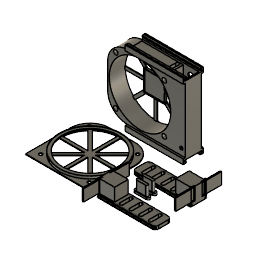
fume_extractor (Autodesk Fusion 360 design; units mm, degrees)
part number: 2026-06-15-13-21-27-474
Autodesk Fusion 360 part; units mm, degrees
(part 1 of 2)
sketch "Sketch1" plane through (0, 0, 0) normal (0, 0, 1) x (1, 0, 0)
  line L0 (-50, -12.5) -> (50, -12.5)
  line L1 (50, -12.5) -> (50, 12.5)
  line L2 (50, 12.5) -> (-50, 12.5)
  line L3 (-50, 12.5) -> (-50, -12.5)
  line L4 (-50, -12.5) -> (50, 12.5) construction
  line L5 (50, -12.5) -> (-50, 12.5) construction
  dimension "d1" = 100
  dimension "d2" = 25
  constraint horizontal L0
  constraint perpendicular L0 L1
  constraint parallel L0 L2
  constraint parallel L1 L3
  constraint coincident L4 origin
  constraint coincident L5 origin
  measures "d1" distance of L1.end L2.end
  measures "d2" distance of L0.end L1.end
extrude "Extrude1" add sketch "Sketch1" along normal blind 120 makes body 1
sketch "Sketch2" plane through (0, 12.5, 0) normal (0, 1, 0) x (-1, 0, 0)
  line L0 (-50, 0) -> (50, 0)
  line L1 (50, 0) -> (50, 120)
  line L2 (50, 120) -> (-50, 120)
  line L3 (-50, 120) -> (-50, 0)
  line L4 (50.0049, 20) -> (-50, 20)
  line L5 (50, 20.0049) -> (50.0049, 20)
  circle A0 centre (0.0025, 70) radius 47.5
  line L6 (6.038, 72.5) -> (47.4366, 72.5)
  line L7 (6.038, 72.5) -> (35.3113, 101.7733)
  line L8 (2.5025, 22.5658) -> (2.5025, 63.9645)
  line L9 (31.7757, 105.3088) -> (2.5025, 76.0355)
  line L10 (-31.7708, 105.3088) -> (-2.4975, 76.0355)
  line L11 (-47.4317, 72.5) -> (-6.0331, 72.5)
  line L12 (-6.0331, 72.5) -> (-35.3063, 101.7733)
  line L13 (47.4366, 67.5) -> (6.038, 67.5)
  line L14 (-6.0331, 67.5) -> (-47.4317, 67.5)
  line L15 (6.038, 67.5) -> (35.3113, 38.2267)
  line L16 (31.7757, 34.6912) -> (2.5025, 63.9645)
  line L17 (-35.3063, 38.2267) -> (-6.0331, 67.5)
  line L18 (-2.4975, 63.9645) -> (-31.7708, 34.6912)
  line L19 (2.5025, 76.0355) -> (2.5025, 117.4342)
  line L20 (-2.4975, 117.4342) -> (-2.4975, 76.0355)
  line L21 (-2.4975, 63.9645) -> (-2.4975, 22.5658)
  point P0 (0.0025, 70)
  point P1 (0.0025, 70)
  point P2 (1.7702, 71.7678)
  dimension "d6" = 20
  dimension "d7" = 95
  constraint coincident L3 L4.end
  constraint parallel L2 L4
  constraint coincident L5 P1
  constraint coincident L1 L5.start
  constraint horizontal L11
  constraint parallel L11 L14
  constraint coincident P1 P0
  constraint parallel L8 L21
  constraint parallel L10 L12
  constraint collinear L20 L21
  constraint collinear L13 L14
  constraint parallel L15 L16
  constraint coincident A0 L12.end
  constraint coincident A0 L10.start
  constraint coincident A0 L11.start
  constraint coincident A0 L14.end
  constraint coincident A0 L19.end
  constraint coincident A0 L20.start
  constraint coincident A0 L9.start
  constraint coincident A0 L7.end
  constraint coincident A0 L6.end
  constraint coincident A0 L13.start
  constraint coincident A0 L15.end
  constraint coincident A0 L16.start
  constraint coincident A0 L21.end
  constraint coincident A0 L8.start
  constraint coincident A0 L17.start
  constraint coincident A0 L18.end
  measures "d6" distance of L0 L4
  measures "d7" diameter of A0
extrude "Extrude2" cut sketch "Sketch2" against normal blind 25 contours A0 L6 L7 | A0 L13 L15 | A0 L9 L19 | A0 L8 L16 | A0 L10 L20 | A0 L18 L21 | A0 L11 L12 | A0 L14 L17 bodies 1
sketch "Sketch7" plane through (0, -12.5, 0) normal (0, -1, 0) x (1, 0, 0)
  line L0 (-50, 0) -> (50, 0)
  line L1 (50, 0) -> (50, 120)
  line L2 (50, 120) -> (-50, 120)
  line L3 (-50, 120) -> (-50, 0)
  line L4 (2.4975, 22.5658) -> (2.4975, 63.9645)
  line L5 (2.4975, 63.9645) -> (31.7708, 34.6912)
  arc A0 (2.4975, 22.5658) -> (31.7708, 34.6912) centre (-0.0025, 70) ccw
  line L6 (-31.7757, 34.6912) -> (-2.5025, 63.9645)
  line L7 (-2.5025, 63.9645) -> (-2.5025, 22.5658)
  arc A1 (-31.7757, 34.6912) -> (-2.5025, 22.5658) centre (-0.0025, 70) ccw
  line L8 (-35.3113, 101.7733) -> (-6.038, 72.5)
  line L9 (-6.038, 72.5) -> (-47.4366, 72.5)
  arc A2 (-35.3113, 101.7733) -> (-47.4366, 72.5) centre (-0.0025, 70) ccw
  line L10 (2.4975, 76.0355) -> (2.4975, 117.4342)
  arc A3 (31.7708, 105.3088) -> (2.4975, 117.4342) centre (-0.0025, 70) ccw
  line L11 (31.7708, 105.3088) -> (2.4975, 76.0355)
  line L12 (-2.5025, 117.4342) -> (-2.5025, 76.0355)
  line L13 (-2.5025, 76.0355) -> (-31.7757, 105.3088)
  arc A4 (-2.5025, 117.4342) -> (-31.7757, 105.3088) centre (-0.0025, 70) ccw
  arc A5 (-47.4366, 67.5) -> (-35.3113, 38.2267) centre (-0.0025, 70) ccw
  line L14 (-47.4366, 67.5) -> (-6.038, 67.5)
  line L15 (-6.038, 67.5) -> (-35.3113, 38.2267)
  line L16 (6.0331, 67.5) -> (47.4317, 67.5)
  arc A6 (35.3063, 38.2267) -> (47.4317, 67.5) centre (-0.0025, 70) ccw
  line L17 (35.3063, 38.2267) -> (6.0331, 67.5)
  arc A7 (47.4317, 72.5) -> (35.3063, 101.7733) centre (-0.0025, 70) ccw
  line L18 (47.4317, 72.5) -> (6.0331, 72.5)
  line L19 (6.0331, 72.5) -> (35.3063, 101.7733)
  circle A8 centre (-0.0025, 70) radius 47.5
  dimension "d36" = 95
  constraint concentric A0 A8
  measures "d36" diameter of A8
extrude "Extrude7" cut sketch "Sketch7" against normal blind 24 contours L4 L5 L6 L7 L8 L9 L10 L11 L12 L13 L14 L15 L16 L17 L18 L19 A8 bodies 1
sketch "Sketch8" plane through (0, 11.5, 0) normal (0, -1, 0) x (1, 0, 0)
  arc A0 (47.4317, 67.5) -> (47.4317, 72.5) centre (-0.0025, 70) ccw
  line L0 (47.4317, 72.5) -> (6.0331, 72.5)
  line L1 (6.0331, 72.5) -> (35.3063, 101.7733)
  arc A1 (35.3063, 101.7733) -> (31.7708, 105.3088) centre (-0.0025, 70) ccw
  line L2 (31.7708, 105.3088) -> (2.4975, 76.0355)
  line L3 (2.4975, 76.0355) -> (2.4975, 117.4342)
  arc A2 (2.4975, 117.4342) -> (-2.5025, 117.4342) centre (-0.0025, 70) ccw
  line L4 (-2.5025, 117.4342) -> (-2.5025, 76.0355)
  line L5 (-2.5025, 76.0355) -> (-31.7757, 105.3088)
  arc A3 (-31.7757, 105.3088) -> (-35.3113, 101.7733) centre (-0.0025, 70) ccw
  line L6 (-35.3113, 101.7733) -> (-6.038, 72.5)
  line L7 (-6.038, 72.5) -> (-47.4366, 72.5)
  arc A4 (-47.4366, 72.5) -> (-47.4366, 67.5) centre (-0.0025, 70) ccw
  line L8 (-47.4366, 67.5) -> (-6.038, 67.5)
  line L9 (-6.038, 67.5) -> (-35.3113, 38.2267)
  arc A5 (-35.3113, 38.2267) -> (-31.7757, 34.6912) centre (-0.0025, 70) ccw
  line L10 (-31.7757, 34.6912) -> (-2.5025, 63.9645)
  line L11 (-2.5025, 63.9645) -> (-2.5025, 22.5658)
  arc A6 (-2.5025, 22.5658) -> (2.4975, 22.5658) centre (-0.0025, 70) ccw
  line L12 (2.4975, 22.5658) -> (2.4975, 63.9645)
  line L13 (2.4975, 63.9645) -> (31.7708, 34.6912)
  arc A7 (31.7708, 34.6912) -> (35.3063, 38.2267) centre (-0.0025, 70) ccw
  line L14 (35.3063, 38.2267) -> (6.0331, 67.5)
  line L15 (6.0331, 67.5) -> (47.4317, 67.5)
  line L16 (16.4975, 86.5) -> (-16.5025, 86.5)
  line L17 (-16.5025, 86.5) -> (-16.5025, 53.5)
  line L18 (-16.5025, 53.5) -> (16.4975, 53.5)
  line L19 (16.4975, 53.5) -> (16.4975, 86.5)
  line L20 (16.4975, 86.5) -> (-16.5025, 53.5) construction
  line L21 (-16.5025, 86.5) -> (16.4975, 53.5) construction
  point P0 (-0.0025, 70)
  dimension "d39" = 33
  dimension "d40" = 33
  constraint horizontal L16
  constraint perpendicular L16 L17
  constraint parallel L16 L18
  constraint parallel L17 L19
  constraint coincident L20 P0
  constraint coincident L21 P0
  constraint coincident P0 A0.centre
  measures "d39" distance of L17.end L18.end
  measures "d40" distance of L16.end L17.end
extrude "Extrude8" add sketch "Sketch8" along normal blind 2 contours L14 L15 L19 | L0 L1 L2 L3 L4 L5 L6 L7 L8 L9 L10 L11 L12 L13 L14 L15 L16 L17 L18 L19 | L0 L1 L19 | L12 L13 L18 | L2 L3 L16 | L10 L11 L18 | L4 L5 L16 | L8 L9 L17 | L6 L7 L17 bodies 1
extrude "Extrude9" add 8 faces at (-13.0143, 11.5, 64.0118) (-13.0143, 11.5, 75.9882) (-5.9906, 11.5, 83.0118) (5.9857, 11.5, 83.0118) (13.0094, 11.5, 75.9882) (13.0094, 11.5, 64.0118) (5.9857, 11.5, 56.9882) (-5.9906, 11.5, 56.9882) along direction (0, 1, 0) blind 1 on bodies 1 bodies 1
sketch "Sketch9" plane through (0, 9.5, 0) normal (0, -1, 0) x (1, 0, 0)
  line L0 (16.4975, 53.5) -> (16.4975, 86.5)
  line L1 (16.4975, 86.5) -> (-16.5025, 86.5)
  line L2 (-16.5025, 86.5) -> (-16.5025, 53.5)
  line L3 (-16.5025, 53.5) -> (16.4975, 53.5)
  line L4 (15.4975, 85.5) -> (-15.5025, 85.5)
  line L5 (-15.5025, 85.5) -> (-15.5025, 54.5)
  line L6 (-15.5025, 54.5) -> (15.4975, 54.5)
  line L7 (15.4975, 54.5) -> (15.4975, 85.5)
  dimension "d45" = 31
  dimension "d46" = 31
  constraint horizontal L4
  constraint perpendicular L4 L5
  constraint parallel L4 L6
  constraint parallel L5 L7
  measures "d45" distance of L5.end L6.end
  measures "d46" distance of L4.end L5.end
extrude "Extrude10" cut sketch "Sketch9" against normal blind 1 contours L4 L5 L6 L7 bodies 1
sketch "Sketch10" plane through (0, 9.5, 0) normal (0, -1, 0) x (1, 0, 0)
  line L0 (-15.5025, 85.5) -> (15.4975, 85.5)
  line L1 (15.4975, 85.5) -> (15.4975, 54.5)
  line L2 (15.4975, 54.5) -> (-15.5025, 54.5)
  line L3 (-15.5025, 54.5) -> (-15.5025, 85.5)
  line L4 (16.4975, 53.5) -> (16.4975, 86.5)
  line L5 (16.4975, 86.5) -> (-16.5025, 86.5)
  line L6 (-16.5025, 86.5) -> (-16.5025, 53.5)
  line L7 (-16.5025, 53.5) -> (16.4975, 53.5)
  line L8 (-1.5, 53.5) -> (-1.5, 54.5)
  line L9 (1.5, 54.5) -> (1.5, 53.5)
  constraint coincident L7 L8.start
  constraint coincident L2 L8.end
  constraint perpendicular L2 L8
  constraint coincident L2 L9.start
  constraint coincident L7 L9.end
  constraint perpendicular L7 L9
extrude "Extrude11" cut sketch "Sketch10" against normal blind 2 contours L2 L7 L8 L9 bodies 1
fillet "Fillet1" radius 30 1 edges at (-50, 0, 120) on bodies 1
fillet "Fillet2" radius 30 1 edges at (50, 0, 120) on bodies 1
sketch "Sketch3" plane through (50, 0, 0) normal (1, 0, 0) x (0, 1, 0)
  line L0 (12.5, 90) -> (-12.5, 90)
  line L1 (-12.5, 90) -> (-12.5, 0)
  line L2 (-12.5, 0) -> (12.5, 0)
  line L3 (12.5, 0) -> (12.5, 90)
  line L4 (-10.5, 20) -> (10.5, 20)
  line L5 (10.5, 20) -> (10.5, 2)
  line L6 (10.5, 2) -> (-10.5, 2)
  line L7 (-10.5, 2) -> (-10.5, 20)
  dimension "d14" = 2
  dimension "d15" = 2
  dimension "d16" = 2
  dimension "d17" = 18
  constraint horizontal L4
  constraint vertical L5
  constraint horizontal L6
  constraint vertical L7
  measures "d14" distance of L3 L5
  measures "d15" distance of L1 L7
  measures "d16" distance of L2 L6
  measures "d17" distance of L4 L6
extrude "Extrude3" cut sketch "Sketch3" against normal blind 98 contours L4 L5 L6 L7 bodies 1
sketch "Sketch4" plane through (0, -10.5, 0) normal (0, 1, 0) x (-1, 0, 0)
  line L0 (-50, 20) -> (-50, 2)
  line L1 (-50, 2) -> (48, 2)
  line L2 (48, 2) -> (48, 20)
  line L3 (48, 20) -> (-50, 20)
  circle A0 centre (-41, 14.5) radius 4.5
  dimension "d20" = 9
  dimension "d21" = 9
  dimension "d22" = 12.5
  measures "d20" diameter of A0
  measures "d21" distance of L0 A0.centre
  measures "d22" distance of L1 A0.centre
extrude "Extrude4" cut sketch "Sketch4" along normal blind 33 contours A0 bodies 1
sketch "Sketch6" plane through (0, 0, 20) normal (0, 0, -1) x (1, 0, 0)
  line L0 (50, -10.5) -> (50, 10.5)
  line L1 (50, 10.5) -> (-48, 10.5)
  line L2 (-48, 10.5) -> (-48, -10.5)
  line L3 (-48, -10.5) -> (50, -10.5)
  circle A0 centre (0, -1.1091) radius 2.5
  dimension "d27" = 5
  measures "d27" diameter of A0
extrude "Extrude6" cut sketch "Sketch6" against normal blind 50 contours A0 bodies 1
sketch "Sketch5" plane through (50, 0, 0) normal (1, 0, 0) x (0, 1, 0)
  line L0 (10.5, 20) -> (10.5, 2)
  line L1 (10.5, 2) -> (-10.5, 2)
  line L2 (-10.5, 2) -> (-10.5, 20)
  line L3 (-10.5, 20) -> (10.5, 20)
  line L4 (12.5, 90) -> (-12.5, 90)
  line L5 (-12.5, 90) -> (-12.5, 0)
  line L6 (-12.5, 0) -> (12.5, 0)
  line L7 (12.5, 0) -> (12.5, 90)
  line L8 (10.5, 20) -> (-10.5, 20)
  line L9 (-10.5, 20) -> (-10.5, 26)
  line L10 (-10.5, 26) -> (10.5, 26)
  line L11 (10.5, 26) -> (10.5, 20)
  constraint perpendicular L8 L9
  constraint parallel L8 L10
  constraint parallel L9 L11
  constraint coincident L2.end L3.start
  constraint perpendicular L2 L8
  constraint coincident L0.start L3.end
extrude "Extrude5" cut sketch "Sketch5" against normal blind 20 contours L3 L8 L9 L10 L11 bodies 1
sketch "Sketch12" plane through (0, -12.5, 0) normal (0, -1, 0) x (1, 0, 0)
  circle A0 centre (-0.0025, 70) radius 47.5
  arc A1 (50, 90) -> (20, 120) centre (20, 90) ccw
  line L0 (20, 120) -> (-20, 120)
  arc A2 (-20, 120) -> (-50, 90) centre (-20, 90) ccw
  line L1 (-50, 90) -> (-50, 0)
  line L2 (-50, 0) -> (50, 0)
  line L3 (50, 0) -> (50, 90)
  circle A3 centre (-40, 6) radius 2.5
  dimension "d54" = 5
  measures "d54" diameter of A3
extrude "Extrude13" cut sketch "Sketch12" against normal blind 2 contours A3 bodies 1
sketch "Sketch13" plane through (0, -12.5, 0) normal (0, -1, 0) x (1, 0, 0)
  circle A0 centre (-40, 6) radius 2.5
  circle A1 centre (-0.0025, 70) radius 47.5
  arc A2 (50, 90) -> (20, 120) centre (20, 90) ccw
  line L0 (20, 120) -> (-20, 120)
  arc A3 (-20, 120) -> (-50, 90) centre (-20, 90) ccw
  line L1 (-50, 90) -> (-50, 0)
  line L2 (-50, 0) -> (50, 0)
  line L3 (50, 0) -> (50, 90)
  line L4 (0, 120) -> (0, 117.5)
  circle A4 centre (37.5, 107.5005) radius 3.5
  circle A5 centre (-37.5, 107.5005) radius 3.5
  circle A6 centre (37.5, 32.5005) radius 3.5
  circle A7 centre (-37.5, 32.5005) radius 3.5
  line L5 (-37.5, 107.5005) -> (37.5, 107.5005)
  line L6 (37.5, 107.5005) -> (37.5, 32.5005)
  line L7 (37.5, 32.5005) -> (-37.5, 32.5005)
  line L8 (-37.5, 32.5005) -> (-37.5, 107.5005)
  dimension "d59" = 75
  dimension "d63" = 75
  dimension "d64" = 37.5
  dimension "d67" = 7
  dimension "d68" = 7
  dimension "d69" = 7
  dimension "d70" = 7
  dimension "d71" = 75
  constraint midpoint L0 L4.start
  constraint perpendicular L0 L4
  constraint coincident A1 L4.end
  constraint coincident A5.centre L5.start
  constraint coincident A4.centre L5.end
  constraint horizontal L5
  constraint coincident A6.centre L6.end
  constraint perpendicular L5 L6
  constraint coincident A7.centre L7.end
  constraint perpendicular L6 L7
  measures "d59" distance of A4.centre A5.centre
  measures "d63" horizontal distance of A6.centre A7.centre
  measures "d64" distance of L4 A5.centre
  measures "d67" diameter of A4
  measures "d68" diameter of A5
  measures "d69" diameter of A6
  measures "d70" diameter of A7
  measures "d71" distance of A5.centre A7.centre
extrude "Extrude14" cut sketch "Sketch13" against normal blind 6 contours A4 L5 L6 | A4 L5 L6 | A6 L6 L7 | A6 L6 L7 | A5 L5 L8 | A5 L5 L8 | A7 L7 L8 | A7 L7 L8 bodies 1
sketch "Sketch14" plane through (0, 0, 0) normal (0, 0, 1) x (1, 0, 0)
  line L0 (20, 50) -> (-20, 50)
  line L1 (-50, 20) -> (-50, -50)
  line L2 (-50, -50) -> (50, -50)
  line L3 (50, -50) -> (50, 20)
  arc A0 (-20, 50) -> (-50, 20) centre (-20, 20) ccw
  arc A1 (50, 20) -> (20, 50) centre (20, 20) ccw
  circle A2 centre (0, 0) radius 47.5
  line L4 (-50, 50) -> (-41.2132, 41.2132) construction
  line L5 (50, 50) -> (41.2132, 41.2132) construction
  circle A3 centre (-37.7911, 36.5) radius 2.5
  circle A4 centre (37.2089, 36.5) radius 2.5
  circle A5 centre (-37.7911, -38.5) radius 2.5
  circle A6 centre (37.2089, -38.5) radius 2.5
  dimension "d72" = 100
  dimension "d73" = 100
  dimension "d74" = 30
  dimension "d75" = 30
  dimension "d76" = 95
  dimension "d81" = 75
  dimension "d82" = 75
  dimension "d84" = 50
  dimension "d85" = 5
  dimension "d86" = 5
  dimension "d87" = 5
  dimension "d88" = 5
  constraint horizontal L0
  constraint perpendicular L0 L1
  constraint parallel L0 L2
  constraint parallel L1 L3
  constraint coincident A2.centre origin
  constraint coincident L4.start L0
  constraint coincident L4.start L1
  constraint tangent L0 A0
  constraint tangent L1 A0
  constraint coincident L5.start L0
  constraint coincident L5.start L3
  constraint tangent L0 A1
  constraint tangent L3 A1
  constraint coincident A0 L4.end
  constraint coincident A1 L5.end
  measures "d72" distance of L1.end L2.end
  measures "d73" distance of L4.start L1.end
  measures "d74" radius of A0
  measures "d75" radius of A1
  measures "d76" diameter of A2
  measures "d81" distance of A3.centre A4.centre
  measures "d82" vertical distance of A3.centre A5.centre
  measures "d84" distance of L0 A2.centre
  measures "d85" diameter of A3
  measures "d86" diameter of A4
  measures "d87" diameter of A5
  measures "d88" diameter of A6
extrude "Extrude15" add sketch "Sketch14" along normal blind 1 separate body makes body 2
sketch "Sketch15" plane through (0, 0, 0) normal (0, 0, 1) x (1, 0, 0)
  circle A0 centre (0, 0) radius 46.5
  circle A1 centre (0, 0) radius 47.5
  dimension "d91" = 93
  dimension "d92" = 95
  constraint coincident A0.centre A1.centre
  constraint concentric A0 A1
  measures "d91" diameter of A0
  measures "d92" diameter of A1
extrude "Extrude16" add sketch "Sketch15" along normal blind 5 bodies 2
sketch "Sketch16" plane through (0, 0, 0) normal (0, 0, 1) x (1, 0, 0)
  circle A0 centre (0, 0) radius 45
  circle A1 centre (0, 0) radius 46.5
  dimension "d95" = 90
  dimension "d96" = 93
  constraint coincident A0.centre A1.centre
  constraint concentric A0 A1
  measures "d95" diameter of A0
  measures "d96" diameter of A1
extrude "Extrude17" add sketch "Sketch16" along normal blind 1 bodies 2
sketch "Sketch17" plane through (0, 0, 5) normal (0, 0, 1) x (-1, 0, 0)
  circle A0 centre (0, 0) radius 46.5
  circle A1 centre (0, 0) radius 47.5
  circle A2 centre (0, 0) radius 42.5
  circle A3 centre (0.5775, 0) radius 47.0775
  dimension "d99" = 85
  constraint concentric A0 A2
  constraint tangent A0 A3
  measures "d99" diameter of A2
extrude "Extrude18" add sketch "Sketch17" against normal blind 1 contours A0 bodies 2
sketch "Sketch18" plane through (0, 0, 0) normal (0, 0, 1) x (1, 0, 0)
  line L0 (-33.5384, 30.0029) -> (-6.0355, 2.5)
  line L1 (6.0355, 2.5) -> (33.5384, 30.0029)
  line L2 (30.0029, 33.5384) -> (2.5, 6.0355)
  line L3 (6.0355, -2.5) -> (33.5384, -30.0029)
  line L4 (30.0029, -33.5384) -> (2.5, -6.0355)
  line L5 (-30.0029, -33.5384) -> (-2.5, -6.0355)
  line L6 (-6.0355, -2.5) -> (-33.5384, -30.0029)
  line L7 (-2.5, 6.0355) -> (-30.0029, 33.5384)
  line L8 (44.9305, 2.5) -> (6.0355, 2.5)
  line L9 (-6.0355, 2.5) -> (-44.9305, 2.5)
  line L10 (-44.9305, -2.5) -> (-6.0355, -2.5)
  line L11 (6.0355, -2.5) -> (44.9305, -2.5)
  line L12 (2.5, 6.0355) -> (2.5, 44.9305)
  line L13 (2.5, -44.9305) -> (2.5, -6.0355)
  line L14 (-2.5, 44.9305) -> (-2.5, 6.0355)
  line L15 (-2.5, -6.0355) -> (-2.5, -44.9305)
  arc A0 (-44.9305, 2.5) -> (-44.9305, -2.5) centre (0, 0) ccw
  arc A1 (-30.0029, 33.5384) -> (-33.5384, 30.0029) centre (0, 0) ccw
  arc A2 (2.5, 44.9305) -> (-2.5, 44.9305) centre (0, 0) ccw
  arc A3 (33.5384, 30.0029) -> (30.0029, 33.5384) centre (0, 0) ccw
  arc A4 (44.9305, -2.5) -> (44.9305, 2.5) centre (0, 0) ccw
  arc A5 (30.0029, -33.5384) -> (33.5384, -30.0029) centre (0, 0) ccw
  arc A6 (-33.5384, -30.0029) -> (-30.0029, -33.5384) centre (0, 0) ccw
  arc A7 (-2.5, -44.9305) -> (2.5, -44.9305) centre (0, 0) ccw
  constraint horizontal L10
  constraint parallel L8 L11
  constraint coincident A0.centre A1.centre
  constraint parallel L13 L15
  constraint parallel L0 L7
  constraint parallel L1 L2
  constraint parallel L3 L4
  constraint collinear L8 L9
  constraint collinear L10 L11
  constraint collinear L14 L15
  constraint concentric A0 A6
  constraint concentric A1 A2
  constraint concentric A2 A3
  constraint concentric A3 A4
  constraint concentric A4 A5
  constraint concentric A5 A7
  constraint concentric A6 A7
extrude "Extrude19" add sketch "Sketch18" along normal blind 1 bodies 2
move_body "Move2" bodies 2 to x (1, 0, 0) y (0, 1, 0) z (0, 0, 1) at (-1.2204, -73.9859, 0)
sketch "Sketch19" plane through (0, 0, 0) normal (0, 0, 1) x (1, 0, 0)
  line L0 (51.3826, -12.4971) -> (56.3826, -12.4971)
  line L1 (56.3826, -12.4971) -> (56.3826, 12.5029)
  line L2 (56.3826, 12.5029) -> (51.3826, 12.5029)
  line L3 (51.3826, 12.5029) -> (51.3826, -12.4971)
  dimension "d108" = 5
  dimension "d113" = 25
  constraint horizontal L0
  constraint vertical L1
  constraint horizontal L2
  constraint vertical L3
  measures "d108" distance of L0.start L0.end
  measures "d113" distance of L0.end L1.end
extrude "Extrude20" add sketch "Sketch19" along normal blind 90 separate body makes body 3
sketch "Sketch21" plane through (56.3826, 0, 0) normal (1, 0, 0) x (0, 1, 0)
  line L0 (-12.4971, 0) -> (12.5029, 0)
  line L1 (12.5029, 0) -> (12.5029, 90)
  line L2 (12.5029, 90) -> (-12.4971, 90)
  line L3 (-12.4971, 90) -> (-12.4971, 0)
  line L4 (7.5, 80) -> (-7.5, 80)
  line L5 (-7.5, 75) -> (7.5, 75)
  line L6 (7.5, 65) -> (-7.5, 65)
  line L7 (-7.5, 60) -> (7.5, 60)
  line L8 (7.5, 50) -> (-7.5, 50)
  line L9 (-7.5, 45) -> (7.5, 45)
  line L10 (7.5, 35) -> (-7.5, 35)
  line L11 (-7.5, 30) -> (7.5, 30)
  arc A0 (7.5, 75) -> (7.5, 80) centre (7.5, 77.5) ccw
  arc A1 (-7.5, 80) -> (-7.5, 75) centre (-7.5, 77.5) ccw
  arc A2 (-7.5, 65) -> (-7.5, 60) centre (-7.5, 62.5) ccw
  arc A3 (7.5, 60) -> (7.5, 65) centre (7.5, 62.5) ccw
  arc A4 (-7.5, 50) -> (-7.5, 45) centre (-7.5, 47.5) ccw
  arc A5 (7.5, 45) -> (7.5, 50) centre (7.5, 47.5) ccw
  arc A6 (-7.5, 35) -> (-7.5, 30) centre (-7.5, 32.5) ccw
  arc A7 (7.5, 30) -> (7.5, 35) centre (7.5, 32.5) ccw
  dimension "d116" = 10
  dimension "d119" = 10
  dimension "d124" = 10
  dimension "d125" = 10
  dimension "d126" = 2.5
  dimension "d127" = 2.5
  dimension "d128" = 2.5
  constraint horizontal L4
  constraint parallel L4 L5
  constraint horizontal L6
  constraint parallel L6 L7
  constraint horizontal L8
  constraint parallel L8 L9
  constraint horizontal L10
  constraint parallel L10 L11
  constraint tangent L4 A0
  constraint tangent L5 A0
  constraint tangent L6 A2
  constraint tangent L7 A2
  constraint tangent L6 A3
  constraint tangent L7 A3
  constraint tangent L8 A4
  constraint tangent L9 A4
  constraint equal A2 A4
  constraint tangent L8 A5
  constraint tangent L9 A5
  constraint tangent L10 A6
  constraint tangent L11 A6
  constraint equal A2 A6
  constraint tangent L10 A7
  constraint tangent L11 A7
  measures "d116" distance of L2 L4
  measures "d119" distance of L5 L6
  measures "d124" distance of L7 L8
  measures "d125" distance of L9 L10
  measures "d126" radius of A0
  measures "d127" radius of A1
  measures "d128" radius of A2
extrude "Extrude22" cut sketch "Sketch21" against normal blind 5 contours L4 L5 A0 A1 | L6 L7 A2 A3 | L8 L9 A4 A5 | L10 L11 A6 A7 bodies 3
sketch "Sketch22" plane through (50, 0, 0) normal (1, 0, 0) x (0, 1, 0)
  line L0 (12.5, 90) -> (-12.5, 90)
  line L1 (-12.5, 90) -> (-12.5, 0)
  line L2 (-12.5, 0) -> (12.5, 0)
  line L3 (12.5, 0) -> (12.5, 90)
  line L4 (-10.5, 2) -> (-10.5, 26)
  line L5 (-10.5, 26) -> (10.5, 26)
  line L6 (10.5, 26) -> (10.5, 2)
  line L7 (10.5, 2) -> (-10.5, 2)
  line L8 (7.5, 34.5) -> (-7.5, 34.5)
  line L9 (-7.5, 29.5) -> (7.5, 29.5)
  arc A0 (7.5, 29.5) -> (7.5, 34.5) centre (7.5, 32) ccw
  arc A1 (-7.5, 34.5) -> (-7.5, 29.5) centre (-7.5, 32) ccw
  dimension "d133" = 2.5
  constraint horizontal L8
  constraint parallel L8 L9
  constraint tangent L8 A1
  constraint tangent L9 A1
  constraint equal A0 A1
  measures "d133" radius of A0
extrude "Extrude23" cut sketch "Sketch22" against normal blind 7 contours L8 L9 A0 A1 bodies 1
fillet "Fillet3" radius 5 1 edges at (53.8826, -12.4971, 90) on bodies 3
fillet "Fillet4" radius 5 1 edges at (53.8826, 12.5029, 90) on bodies 3
sketch "Sketch23" plane through (56.3826, 0, 0) normal (1, 0, 0) x (0, 1, 0)
  line L0 (-7.5, 65) -> (7.5, 65)
  arc A0 (7.5, 60) -> (7.5, 65) centre (7.5, 62.5) ccw
  line L1 (7.5, 60) -> (-7.5, 60)
  arc A1 (-7.5, 65) -> (-7.5, 60) centre (-7.5, 62.5) ccw
  line L2 (-7.5, 50) -> (7.5, 50)
  arc A2 (7.5, 45) -> (7.5, 50) centre (7.5, 47.5) ccw
  line L3 (7.5, 45) -> (-7.5, 45)
  arc A3 (-7.5, 50) -> (-7.5, 45) centre (-7.5, 47.5) ccw
  line L4 (7.5, 75) -> (-7.5, 75)
  arc A4 (-7.5, 80) -> (-7.5, 75) centre (-7.5, 77.5) ccw
  line L5 (-7.5, 80) -> (7.5, 80)
  arc A5 (7.5, 75) -> (7.5, 80) centre (7.5, 77.5) ccw
  line L6 (-7.5, 35) -> (7.5, 35)
  arc A6 (7.5, 30) -> (7.5, 35) centre (7.5, 32.5) ccw
  line L7 (7.5, 30) -> (-7.5, 30)
  arc A7 (-7.5, 35) -> (-7.5, 30) centre (-7.5, 32.5) ccw
  arc A8 (12.5029, 85) -> (7.5029, 90) centre (7.5029, 85) ccw
  line L8 (7.5029, 90) -> (-7.4971, 90)
  arc A9 (-7.4971, 90) -> (-12.4971, 85) centre (-7.4971, 85) ccw
  line L9 (-12.4971, 85) -> (-12.4971, 0)
  line L10 (-12.4971, 0) -> (12.5029, 0)
  line L11 (12.5029, 0) -> (12.5029, 85)
  line L12 (-12.4971, 0) -> (12.5029, 0)
  line L13 (12.5029, 0) -> (12.5029, 25)
  line L14 (12.5029, 25) -> (-12.4971, 25)
  line L15 (-12.4971, 25) -> (-12.4971, 0)
  dimension "d140" = 25
  constraint perpendicular L12 L13
  constraint parallel L12 L14
  constraint parallel L13 L15
  constraint coincident L10.end L11.start
  constraint perpendicular L11 L12
  constraint coincident L9.end L10.start
  measures "d140" distance of L9.end L14.end
extrude "Extrude24" add sketch "Sketch23" along normal blind 20 contours L9 L10 L11 L12 L13 L14 L15 bodies 3
sketch "Sketch28" plane through (76.3826, 0, 0) normal (1, 0, 0) x (0, 1, 0)
  line L0 (-12.4971, 25) -> (-12.4971, 0)
  line L1 (-12.4971, 0) -> (12.5029, 0)
  line L2 (12.5029, 0) -> (12.5029, 25)
  line L3 (12.5029, 25) -> (-12.4971, 25)
  line L4 (-10.4971, 25) -> (-10.4971, 2)
  line L5 (-10.4971, 2) -> (10.5029, 2)
  line L6 (10.5029, 2) -> (10.5029, 25)
  constraint coincident L3 L4.start
  constraint perpendicular L1 L4
  constraint perpendicular L2 L5
  constraint coincident L3 L6.end
  constraint perpendicular L3 L6
extrude "Extrude29" cut sketch "Sketch28" against normal blind 20 contours L0 L1 L2 L3 L4 L5 L6 bodies 3
sketch "Sketch29" plane through (56.3826, 0, 0) normal (1, 0, 0) x (0, 1, 0)
  line L0 (12.5029, 0) -> (12.5029, 85)
  line L1 (7.5029, 90) -> (-7.4971, 90)
  arc A0 (-7.4971, 90) -> (-12.4971, 85) centre (-7.4971, 85) ccw
  line L2 (-12.4971, 85) -> (-12.4971, 0)
  line L3 (-12.4971, 0) -> (12.5029, 0)
  line L4 (10.5029, 2) -> (-10.4971, 2)
  line L5 (-10.4971, 2) -> (-10.4971, 25)
  line L6 (-10.4971, 25) -> (10.5029, 25)
  line L7 (-7.5, 65) -> (7.5, 65)
  arc A1 (7.5, 60) -> (7.5, 65) centre (7.5, 62.5) ccw
  line L8 (7.5, 60) -> (-7.5, 60)
  arc A2 (-7.5, 65) -> (-7.5, 60) centre (-7.5, 62.5) ccw
  line L9 (-7.5, 50) -> (7.5, 50)
  arc A3 (7.5, 45) -> (7.5, 50) centre (7.5, 47.5) ccw
  line L10 (7.5, 45) -> (-7.5, 45)
  arc A4 (-7.5, 50) -> (-7.5, 45) centre (-7.5, 47.5) ccw
  line L11 (7.5, 75) -> (-7.5, 75)
  arc A5 (-7.5, 80) -> (-7.5, 75) centre (-7.5, 77.5) ccw
  line L12 (-7.5, 80) -> (7.5, 80)
  arc A6 (7.5, 75) -> (7.5, 80) centre (7.5, 77.5) ccw
  line L13 (-7.5, 35) -> (7.5, 35)
  arc A7 (7.5, 30) -> (7.5, 35) centre (7.5, 32.5) ccw
  line L14 (7.5, 30) -> (-7.5, 30)
  arc A8 (-7.5, 35) -> (-7.5, 30) centre (-7.5, 32.5) ccw
  line L15 (-0.4971, 2) -> (-0.4971, 0)
  line L16 (0.5029, 2) -> (0.5029, 0)
  arc A9 (12.5029, 85) -> (7.5029, 90) centre (7.5029, 85) ccw
  line L17 (10.5029, 25) -> (10.5029, 2)
  dimension "d169" = 12
  dimension "d170" = 12
  constraint coincident L4 L15.start
  constraint coincident L3 L15.end
  constraint perpendicular L3 L15
  constraint coincident L4 L16.start
  constraint coincident L3 L16.end
  constraint perpendicular L3 L16
  measures "d169" distance of L0 L16
  measures "d170" distance of L2 L15
extrude "Extrude30" add sketch "Sketch29" along normal blind 20 contours L3 L4 L15 L16 bodies 3
sketch "Sketch30" plane through (56.3826, 0, 0) normal (1, 0, 0) x (0, 1, 0)
  line L0 (-7.5, 35) -> (7.5, 35)
  arc A0 (7.5, 30) -> (7.5, 35) centre (7.5, 32.5) ccw
  line L1 (7.5, 30) -> (-7.5, 30)
  arc A1 (-7.5, 35) -> (-7.5, 30) centre (-7.5, 32.5) ccw
  line L2 (7.5, 75) -> (-7.5, 75)
  arc A2 (-7.5, 80) -> (-7.5, 75) centre (-7.5, 77.5) ccw
  line L3 (-7.5, 80) -> (7.5, 80)
  arc A3 (7.5, 75) -> (7.5, 80) centre (7.5, 77.5) ccw
  line L4 (-7.5, 50) -> (7.5, 50)
  arc A4 (7.5, 45) -> (7.5, 50) centre (7.5, 47.5) ccw
  line L5 (7.5, 45) -> (-7.5, 45)
  arc A5 (-7.5, 50) -> (-7.5, 45) centre (-7.5, 47.5) ccw
  line L6 (-7.5, 65) -> (7.5, 65)
  arc A6 (7.5, 60) -> (7.5, 65) centre (7.5, 62.5) ccw
  line L7 (7.5, 60) -> (-7.5, 60)
  arc A7 (-7.5, 65) -> (-7.5, 60) centre (-7.5, 62.5) ccw
  line L8 (-0.4971, 2) -> (-10.4971, 2)
  line L9 (-10.4971, 2) -> (-10.4971, 25)
  line L10 (-10.4971, 25) -> (10.5029, 25)
  line L11 (0.5029, 2) -> (0.5029, 0)
  line L12 (0.5029, 0) -> (12.5029, 0)
  line L13 (12.5029, 0) -> (12.5029, 85)
  line L14 (7.5029, 90) -> (-7.4971, 90)
  arc A8 (-7.4971, 90) -> (-12.4971, 85) centre (-7.4971, 85) ccw
  line L15 (-12.4971, 85) -> (-12.4971, 0)
  line L16 (12.5029, 0) -> (0.5029, 0)
  line L17 (0.5029, 0) -> (0.5029, 2)
  line L18 (0.5029, 2) -> (12.5029, 2)
  line L19 (12.5029, 2) -> (12.5029, 0)
  line L20 (0.5039, 1.5) -> (12.0029, 1.5)
  line L21 (12.0029, 1.5) -> (12.0029, 0.5)
  line L22 (12.0029, 0.5) -> (0.5039, 0.5)
  line L23 (0.5039, 0.5) -> (0.5039, 1.5)
  line L24 (-0.4971, 0) -> (-0.4971, 2)
  line L25 (10.5029, 25) -> (10.5029, 2)
  line L26 (10.5029, 2) -> (0.5029, 2)
  arc A9 (12.5029, 85) -> (7.5029, 90) centre (7.5029, 85) ccw
  line L27 (-12.4971, 0) -> (-0.4971, 0)
  dimension "d173" = 0.5
  dimension "d174" = 0.5
  dimension "d175" = 0.001
  dimension "d176" = 0.5
  constraint horizontal L16
  constraint vertical L17
  constraint horizontal L18
  constraint vertical L19
  constraint coincident L11.start L17.end
  constraint coincident L12.end L13.start
  constraint horizontal L20
  constraint vertical L21
  constraint horizontal L22
  constraint vertical L23
  measures "d173" distance of L16 L22
  measures "d174" distance of L18 L20
  measures "d175" distance of L17 L23
  measures "d176" distance of L19 L20.end
extrude "Extrude31" add sketch "Sketch30" along normal blind 20 contours L11 L12 L13 L16 L17 L18 L19 L26 bodies 3
sketch "Sketch31" plane through (0, 12.5029, 0) normal (0, 1, 0) x (-1, 0, 0)
  line L0 (-76.3826, 0) -> (-51.3826, 0)
  line L1 (-51.3826, 0) -> (-51.3826, 85)
  line L2 (-56.3826, 85) -> (-56.3826, 2)
  line L3 (-76.3826, 2) -> (-76.3826, 0)
  line L4 (-75.8826, 2) -> (-56.8826, 2)
  line L5 (-56.8826, 2) -> (-56.8826, 0)
  line L6 (-56.8826, 0) -> (-75.8826, 0)
  line L7 (-75.8826, 0) -> (-75.8826, 2)
  line L8 (-51.3826, 85) -> (-56.3826, 85)
  line L9 (-56.3826, 2) -> (-76.3826, 2)
  dimension "d179" = 0.5
  dimension "d180" = 5.5
  constraint horizontal L4
  constraint vertical L5
  constraint horizontal L6
  constraint vertical L7
  constraint coincident L0 L5.end
  measures "d179" distance of L3 L7
  measures "d180" distance of L1 L5
extrude "Extrude32" cut sketch "Sketch31" against normal blind 12 contours L0 L4 L5 L6 L7 L9 bodies 3
extrude "Extrude33" add 1 faces at (69.5492, 0.5029, 0.6667) along direction (0, 1, 0) blind 0.001 on bodies 3 bodies 3
extrude "Extrude34" add 1 faces at (69.5492, 0.5039, 0.8333) along direction (0, 1, 0) blind 5 on bodies 3 bodies 3
sketch "Sketch33" plane through (56.3826, 0, 0) normal (1, 0, 0) x (0, 1, 0)
  line L0 (12.5029, 2) -> (12.5029, 85)
  line L1 (-12.4971, 0) -> (-0.4971, 0)
  line L2 (-0.4971, 0) -> (-0.4971, 2)
  line L3 (-0.4971, 2) -> (-10.4971, 2)
  line L4 (-0.4981, 0.5) -> (-11.9971, 0.5)
  line L5 (-11.9971, 0.5) -> (-11.9971, 1.5)
  line L6 (-11.9971, 1.5) -> (-0.4981, 1.5)
  line L7 (-0.4981, 1.5) -> (-0.4981, 0.5)
  line L8 (-10.4971, 2) -> (-12.4971, 2)
  line L9 (10.5029, 2) -> (12.5029, 2)
  arc A0 (12.5029, 85) -> (7.5029, 90) centre (7.5029, 85) ccw
  line L10 (7.5029, 90) -> (-7.4971, 90)
  arc A1 (-7.4971, 90) -> (-12.4971, 85) centre (-7.4971, 85) ccw
  line L11 (-12.4971, 85) -> (-12.4971, 0)
  line L12 (-10.4971, 2) -> (-10.4971, 25)
  line L13 (-10.4971, 25) -> (10.5029, 25)
  line L14 (10.5029, 25) -> (10.5029, 2)
  line L15 (-7.5, 65) -> (7.5, 65)
  arc A2 (7.5, 60) -> (7.5, 65) centre (7.5, 62.5) ccw
  line L16 (7.5, 60) -> (-7.5, 60)
  arc A3 (-7.5, 65) -> (-7.5, 60) centre (-7.5, 62.5) ccw
  line L17 (-7.5, 50) -> (7.5, 50)
  arc A4 (7.5, 45) -> (7.5, 50) centre (7.5, 47.5) ccw
  line L18 (7.5, 45) -> (-7.5, 45)
  arc A5 (-7.5, 50) -> (-7.5, 45) centre (-7.5, 47.5) ccw
  line L19 (7.5, 75) -> (-7.5, 75)
  arc A6 (-7.5, 80) -> (-7.5, 75) centre (-7.5, 77.5) ccw
  line L20 (-7.5, 80) -> (7.5, 80)
  arc A7 (7.5, 75) -> (7.5, 80) centre (7.5, 77.5) ccw
  line L21 (-7.5, 35) -> (7.5, 35)
  arc A8 (7.5, 30) -> (7.5, 35) centre (7.5, 32.5) ccw
  line L22 (7.5, 30) -> (-7.5, 30)
  arc A9 (-7.5, 35) -> (-7.5, 30) centre (-7.5, 32.5) ccw
  dimension "d188" = 0.5
  dimension "d190" = 0.5
  dimension "d191" = 0.001
  constraint horizontal L4
  constraint vertical L5
  constraint horizontal L6
  constraint vertical L7
  constraint coincident L3.end L8.start
  measures "d188" distance of L3 L6
  measures "d190" distance of L1 L4
  measures "d191" distance of L2 L7
extrude "Extrude35" add sketch "Sketch33" along normal blind 20 contours L1 L2 L3 L8 L11 bodies 3
sketch "Sketch34" plane through (0, -12.4971, 0) normal (0, -1, 0) x (1, 0, 0)
  line L0 (56.3826, 85) -> (51.3826, 85)
  line L1 (51.3826, 85) -> (51.3826, 0)
  line L2 (51.3826, 0) -> (76.3826, 0)
  line L3 (76.3826, 0) -> (76.3826, 2)
  line L4 (56.8826, 2) -> (75.8826, 2)
  line L5 (75.8826, 2) -> (75.8826, 0)
  line L6 (75.8826, 0) -> (56.8826, 0)
  line L7 (56.8826, 0) -> (56.8826, 2)
  line L8 (56.3826, 2) -> (56.3826, 85)
  line L9 (76.3826, 2) -> (56.3826, 2)
  dimension "d194" = 0.5
  dimension "d195" = 5.5
  constraint horizontal L4
  constraint vertical L5
  constraint horizontal L6
  constraint vertical L7
  constraint coincident L2 L5.end
  measures "d194" distance of L3 L5
  measures "d195" distance of L1 L7
extrude "Extrude36" cut sketch "Sketch34" against normal blind 12 contours L2 L4 L5 L6 L7 L9 bodies 3
extrude "Extrude37" add 1 faces at (63.2159, -0.4971, 1.3333) along direction (0, -1, 0) blind 0.001 on bodies 3 bodies 3
extrude "Extrude38" add 1 faces at (63.2159, -0.4981, 1.1667) along direction (0, -1, 0) blind 5 on bodies 3 bodies 3
sketch "Sketch36" plane through (56.8826, 0, 0) normal (1, 0, 0) x (0, 1, 0)
  line L0 (5.5039, 2) -> (5.5039, 1.5)
  line L1 (5.5039, 1.5) -> (12.0029, 1.5)
  line L2 (12.0029, 1.5) -> (12.0029, 0.5)
  line L3 (12.0029, 0.5) -> (5.5039, 0.5)
  line L4 (5.5039, 0.5) -> (5.5039, 0)
  line L5 (5.5039, 0) -> (12.5029, 0)
  line L6 (12.5029, 0) -> (12.5029, 2)
  line L7 (12.5029, 2) -> (10.5029, 2)
  line L8 (10.5029, 2) -> (5.5039, 2)
  line L9 (12.5029, 2) -> (12.5029, 0)
  line L10 (12.5029, 0) -> (35.5029, 0)
  line L11 (35.5029, 0) -> (35.5029, 2)
  line L12 (35.5029, 2) -> (12.5029, 2)
  dimension "d202" = 23
  constraint perpendicular L9 L10
  constraint parallel L9 L11
  constraint parallel L10 L12
  constraint coincident L5.end L6.start
  constraint perpendicular L5 L9
  constraint coincident L6.end L7.start
  measures "d202" distance of L6.end L11.end
extrude "Extrude39" add sketch "Sketch36" along normal blind 18.5 separate body contours L6 L9 L10 L11 L12 makes body 4
extrude "Extrude40" cut 1 faces at (56.8826, 20.1696, 1.3333) along direction (1, 0, 0) blind 0.5 on bodies 4 bodies 4
sketch "Sketch37" plane through (75.3826, 0, 0) normal (1, 0, 0) x (0, 1, 0)
  line L0 (35.5029, 2) -> (12.5029, 2)
  line L1 (12.5029, 2) -> (12.5029, 0)
  line L2 (12.5029, 0) -> (35.5029, 0)
  line L3 (35.5029, 0) -> (35.5029, 2)
  circle A0 centre (13.2529, 1) radius 0.25
  dimension "d207" = 0.5
  dimension "d208" = 1
  dimension "d214" = 0.75
  measures "d207" diameter of A0
  measures "d208" distance of L0 A0.centre
  measures "d214" distance of L1 A0.centre
extrude "Extrude41" add sketch "Sketch37" along normal blind 2 contours A0 bodies 4
sketch "Sketch38" plane through (77.3826, 0, 0) normal (1, 0, 0) x (0, 1, 0)
  circle A0 centre (13.2529, 1) radius 0.25
  circle A1 centre (13.2529, 1) radius 1
  circle A2 centre (13.2529, 1) radius 0.25
  dimension "d211" = 2
  constraint concentric A0 A1
  constraint concentric A1 A2
  measures "d211" diameter of A1
extrude "Extrude42" add sketch "Sketch38" against normal blind 0.5 bodies 3 4
sketch "Sketch39" plane through (57.3826, 0, 0) normal (-1, 0, 0) x (0, -1, 0)
  line L0 (-12.5029, 2) -> (-35.5029, 2)
  line L1 (-35.5029, 2) -> (-35.5029, 0)
  line L2 (-35.5029, 0) -> (-12.5029, 0)
  line L3 (-12.5029, 0) -> (-12.5029, 2)
  circle A0 centre (-13.2529, 1) radius 0.25
  dimension "d215" = 0.5
  dimension "d216" = 0.75
  dimension "d217" = 1
  measures "d215" diameter of A0
  measures "d216" distance of L3 A0.centre
  measures "d217" distance of L0 A0.centre
extrude "Extrude43" add sketch "Sketch39" along normal blind 0.75 contours A0 bodies 4
move_body "Move4" bodies 4 to x (1, 0, 0) y (0, 1, 0) z (0, 0, 1) at (0, -1.8, 0)
extrude "Extrude44" add 1 faces at (69.3826, 33.7029, 0.6667) along direction (0, 1, 0) blind 2 on bodies 4 bodies 4
fillet "Fillet7" radius 1 1 edges at (76.1326, 12.5029, 2) on bodies 3
fillet "Fillet8" radius 1 1 edges at (76.1326, 12.5029, 0) on bodies 3
fillet "Fillet9" radius 1 1 edges at (66.3826, 10.7029, 2) on bodies 4
fillet "Fillet10" radius 1 1 edges at (66.3826, 10.7029, 0) on bodies 4
copy_body "CopyPasteBodies1" bodies 4 makes body 5
move_body "Move5" bodies 5 to x (1, 0, 0) y (0, -1, 0) z (0, 0, -1) at (0, 0.4059, 2)
fillet "Fillet11" radius 1 1 edges at (76.1326, -12.4971, 2) on bodies 3
fillet "Fillet12" radius 1 1 edges at (76.1326, -12.4971, 0) on bodies 3
sketch "Sketch40" plane through (0, 12.5029, 0) normal (0, 1, 0) x (-1, 0, 0)
  line L0 (-56.8826, 2) -> (-56.8826, 0)
  line L1 (-56.8826, 0) -> (-51.3826, 0)
  line L2 (-51.3826, 0) -> (-51.3826, 85)
  line L3 (-51.3826, 85) -> (-56.3826, 85)
  line L4 (-56.3826, 85) -> (-56.3826, 2)
  line L5 (-56.3826, 2) -> (-56.8826, 2)
  line L6 (-55.1, 90.8) -> (-52.6, 90.8)
  line L7 (-52.6, 90.8) -> (-52.6, 0)
  line L8 (-52.6, 0) -> (-55.1, 0)
  line L9 (-55.1, 0) -> (-55.1, 90.8)
  dimension "d234" = 2.5
  constraint perpendicular L6 L7
  constraint parallel L6 L8
  constraint parallel L7 L9
  constraint parallel L3 L6
  measures "d234" distance of L6.start L6.end
extrude "Extrude45" cut sketch "Sketch40" against normal blind 2.4 contours L1 L3 L7 L8 L9 | L3 L6 L7 L9 bodies 3
sketch "Sketch41" plane through (0, -12.4971, 0) normal (0, -1, 0) x (1, 0, 0)
  line L0 (56.8826, 0) -> (56.8826, 2)
  line L1 (56.8826, 2) -> (56.3826, 2)
  line L2 (56.3826, 2) -> (56.3826, 85)
  line L3 (56.3826, 85) -> (51.3826, 85)
  line L4 (51.3826, 85) -> (51.3826, 0)
  line L5 (51.3826, 0) -> (56.8826, 0)
  line L6 (52.5, 0) -> (55, 0)
  line L7 (55, 0) -> (55, 93.2879)
  line L8 (55, 93.2879) -> (52.5, 93.2879)
  line L9 (52.5, 93.2879) -> (52.5, 0)
  constraint perpendicular L6 L7
  constraint parallel L6 L8
  constraint parallel L7 L9
  constraint coincident L5 L6.end
  constraint perpendicular L4 L6
extrude "Extrude46" cut sketch "Sketch41" against normal blind 2.4 contours L3 L5 L6 L7 L9 | L3 L7 L8 L9 bodies 3
move_body "Move6" bodies 4 3 5 to x (1, 0, 0) y (0, 1, 0) z (0, 0, 1) at (-1.0137, -104.5337, 0)
sketch "Sketch43" plane through (50, 0, 0) normal (1, 0, 0) x (0, 1, 0)
  line L0 (7.5, 29.5) -> (-7.5, 29.5)
  arc A0 (-7.5, 34.5) -> (-7.5, 29.5) centre (-7.5, 32) ccw
  line L1 (-7.5, 34.5) -> (7.5, 34.5)
  arc A1 (7.5, 29.5) -> (7.5, 34.5) centre (7.5, 32) ccw
  line L2 (12.5, 90) -> (-12.5, 90)
  line L3 (-12.5, 90) -> (-12.5, 0)
  line L4 (-12.5, 0) -> (12.5, 0)
  line L5 (12.5, 0) -> (12.5, 90)
  line L6 (-10.5, 2) -> (-10.5, 26)
  line L7 (-10.5, 26) -> (10.5, 26)
  line L8 (10.5, 26) -> (10.5, 2)
  line L9 (10.5, 2) -> (-10.5, 2)
  line L10 (10.5, 26) -> (10.5, 90)
  line L11 (-10.5, 26) -> (-10.5, 90)
  constraint coincident L7.end L8.start
  constraint coincident L2 L10.end
  constraint perpendicular L2 L10
  constraint coincident L6.end L7.start
  constraint coincident L2 L11.end
  constraint perpendicular L2 L11
extrude "Extrude47" add sketch "Sketch43" along normal blind 3 contours L2 L3 L4 L5 L6 L8 L9 L10 L11 bodies 1
sketch "Sketch44" plane through (0, 12.5, 0) normal (0, 1, 0) x (-1, 0, 0)
  arc A0 (-35.3063, 101.7733) -> (-47.4317, 72.5) centre (0.0025, 70) ccw
  line L0 (-35.3063, 101.7733) -> (-16.4975, 82.9645)
  line L1 (-16.4975, 82.9645) -> (-16.4975, 72.5)
  line L2 (-16.4975, 72.5) -> (-47.4317, 72.5)
  line L3 (-47.4317, 67.5) -> (-16.4975, 67.5)
  line L4 (-16.4975, 67.5) -> (-16.4975, 57.0355)
  line L5 (-16.4975, 57.0355) -> (-35.3063, 38.2267)
  arc A1 (-47.4317, 67.5) -> (-35.3063, 38.2267) centre (0.0025, 70) ccw
  arc A2 (35.3113, 38.2267) -> (47.4366, 67.5) centre (0.0025, 70) ccw
  line L6 (35.3113, 38.2267) -> (16.5025, 57.0355)
  line L7 (16.5025, 57.0355) -> (16.5025, 67.5)
  line L8 (16.5025, 67.5) -> (47.4366, 67.5)
  line L9 (2.5025, 86.5) -> (2.5025, 117.4342)
  arc A3 (31.7757, 105.3088) -> (2.5025, 117.4342) centre (0.0025, 70) ccw
  line L10 (31.7757, 105.3088) -> (12.9669, 86.5)
  line L11 (12.9669, 86.5) -> (2.5025, 86.5)
  line L12 (-2.4975, 117.4342) -> (-2.4975, 86.5)
  line L13 (-2.4975, 86.5) -> (-12.962, 86.5)
  line L14 (-12.962, 86.5) -> (-31.7708, 105.3088)
  arc A4 (-2.4975, 117.4342) -> (-31.7708, 105.3088) centre (0.0025, 70) ccw
  line L15 (16.5025, 82.9645) -> (35.3113, 101.7733)
  arc A5 (47.4366, 72.5) -> (35.3113, 101.7733) centre (0.0025, 70) ccw
  line L16 (47.4366, 72.5) -> (16.5025, 72.5)
  line L17 (16.5025, 72.5) -> (16.5025, 82.9645)
  line L18 (12.9669, 53.5) -> (31.7757, 34.6912)
  arc A6 (2.5025, 22.5658) -> (31.7757, 34.6912) centre (0.0025, 70) ccw
  line L19 (2.5025, 22.5658) -> (2.5025, 53.5)
  line L20 (2.5025, 53.5) -> (12.9669, 53.5)
  line L21 (-2.4975, 53.5) -> (-2.4975, 22.5658)
  arc A7 (-31.7708, 34.6912) -> (-2.4975, 22.5658) centre (0.0025, 70) ccw
  line L22 (-31.7708, 34.6912) -> (-12.962, 53.5)
  line L23 (-12.962, 53.5) -> (-2.4975, 53.5)
  arc A8 (-20, 120) -> (-50, 90) centre (-20, 90) ccw
  line L24 (-50, 90) -> (-53, 90)
  line L25 (-53, 90) -> (-53, 0)
  line L26 (-53, 0) -> (50, 0)
  line L27 (50, 0) -> (50, 90)
  arc A9 (50, 90) -> (20, 120) centre (20, 90) ccw
  line L28 (20, 120) -> (-20, 120)
  circle A10 centre (-41, 14.5) radius 4.5
  line L29 (-50, 90) -> (-50, 0)
  line L30 (-50, 90) -> (-58, 90)
  line L31 (-58, 90) -> (-58, 0)
  line L32 (-58, 0) -> (-50, 0)
  constraint coincident A8.end L24.start
  constraint coincident L26 L29.end
  constraint tangent A8 L29
  constraint perpendicular L25 L30
  constraint perpendicular L30 L31
  constraint perpendicular L29 L32
extrude "Extrude48" add sketch "Sketch44" along normal blind 3 contours L24 L25 L26 L29 L30 L32 | L25 L30 L31 L32 bodies 1
sketch "Sketch45" plane through (0, 12.5, 0) normal (0, -1, 0) x (1, 0, 0)
  line L0 (53, 90) -> (53, 0)
  line L1 (53, 0) -> (58, 0)
  line L2 (58, 0) -> (58, 90)
  line L3 (58, 90) -> (53, 90)
  line L4 (55.5, 90) -> (57.5, 90)
  line L5 (57.5, 90) -> (57.5, 0)
  line L6 (57.5, 0) -> (55.5, 0)
  line L7 (55.5, 0) -> (55.5, 90)
  dimension "d243" = 2
  constraint perpendicular L4 L5
  constraint parallel L4 L6
  constraint parallel L5 L7
  constraint coincident L3 L4.end
  constraint perpendicular L2 L4
  constraint midpoint L3 L4.start
  measures "d243" distance of L4.start L4.end
extrude "Extrude49" add sketch "Sketch45" along normal blind 2 contours L1 L3 L4 L5 L6 L7 bodies 1
sketch "Sketch46" plane through (0, -12.5, 0) normal (0, -1, 0) x (1, 0, 0)
  arc A0 (50, 90) -> (20, 120) centre (20, 90) ccw
  line L0 (20, 120) -> (-20, 120)
  arc A1 (-20, 120) -> (-50, 90) centre (-20, 90) ccw
  line L1 (-50, 90) -> (-50, 0)
  line L2 (-50, 0) -> (53, 0)
  line L3 (53, 0) -> (53, 90)
  line L4 (53, 90) -> (50, 90)
  circle A2 centre (-0.0025, 70) radius 47.5
  circle A3 centre (-40, 6) radius 2.5
  circle A4 centre (-37.5, 32.5005) radius 3.5
  circle A5 centre (37.5, 32.5005) radius 3.5
  circle A6 centre (-37.5, 107.5005) radius 3.5
  circle A7 centre (37.5, 107.5005) radius 3.5
  line L5 (50, 90) -> (50, 0)
  line L6 (58, 0) -> (58, 90)
  line L7 (58, 90) -> (50, 90)
  line L8 (50, 0) -> (58, 0)
  constraint coincident A0.start L4.end
  constraint coincident L2 L5.end
  constraint tangent A0 L5
  constraint perpendicular L2 L6
  constraint perpendicular L5 L7
  constraint perpendicular L6 L8
extrude "Extrude50" add sketch "Sketch46" along normal blind 3 contours L2 L3 L4 L5 L7 L8 | L3 L6 L7 L8 bodies 1
sketch "Sketch47" plane through (0, -12.5, 0) normal (0, 1, 0) x (-1, 0, 0)
  line L0 (-53, 0) -> (-53, 90)
  line L1 (-53, 90) -> (-58, 90)
  line L2 (-58, 90) -> (-58, 0)
  line L3 (-58, 0) -> (-53, 0)
  line L4 (-57.5, 90) -> (-55.5, 90)
  line L5 (-55.5, 90) -> (-55.5, 0)
  line L6 (-55.5, 0) -> (-57.5, 0)
  line L7 (-57.5, 0) -> (-57.5, 90)
  dimension "d248" = 0.5
  dimension "d249" = 2
  constraint perpendicular L4 L5
  constraint parallel L4 L6
  constraint parallel L5 L7
  constraint coincident L1 L4.end
  constraint coincident L1 L4.start
  measures "d248" distance of L2 L7
  measures "d249" distance of L5 L7
extrude "Extrude51" add sketch "Sketch47" along normal blind 2 contours L1 L3 L4 L5 L6 L7 bodies 1
sketch "Sketch48" plane through (-50, 0, 0) normal (-1, 0, 0) x (0, -1, 0)
  line L0 (12.5, 90) -> (-12.5, 90)
  line L1 (-12.5, 90) -> (-12.5, 0)
  line L2 (-12.5, 0) -> (12.5, 0)
  line L3 (12.5, 0) -> (12.5, 90)
  line L4 (7.5, 35) -> (-7.5, 35)
  line L5 (-7.5, 30) -> (7.5, 30)
  arc A0 (7.5, 30) -> (7.5, 35) centre (7.5, 32.5) ccw
  arc A1 (-7.5, 35) -> (-7.5, 30) centre (-7.5, 32.5) ccw
  dimension "d256" = 2.5
  constraint horizontal L4
  constraint horizontal L5
  constraint tangent L4 A0
  constraint tangent L5 A0
  constraint tangent L4 A1
  constraint tangent L5 A1
  measures "d256" radius of A0
extrude "Extrude52" cut sketch "Sketch48" against normal blind 7 contours L4 L5 A0 A1 bodies 1
copy_body "CopyPasteBodies2" bodies 3 4 5 makes body 6 makes body 7 makes body 8
move_body "Move8" bodies 6 7 8 to x (1, 0, 0) y (0, 1, 0) z (0, 0, 1) at (21.208, 50.2635, 0)
sketch "Sketch49" plane through (-50, 0, 0) normal (-1, 0, 0) x (0, -1, 0)
  line L0 (7.5, 30) -> (-7.5, 30)
  arc A0 (-7.5, 35) -> (-7.5, 30) centre (-7.5, 32.5) ccw
  line L1 (-7.5, 35) -> (7.5, 35)
  arc A1 (7.5, 30) -> (7.5, 35) centre (7.5, 32.5) ccw
  line L2 (12.5, 90) -> (-12.5, 90)
  line L3 (-12.5, 90) -> (-12.5, 0)
  line L4 (-12.5, 0) -> (12.5, 0)
  line L5 (12.5, 0) -> (12.5, 90)
  line L6 (12.5, 90) -> (10.5, 90)
  line L7 (10.5, 90) -> (10.5, 0)
  line L8 (10.5, 0) -> (12.5, 0)
  line L9 (12.5, 0) -> (12.5, 90)
  dimension "d259" = 2
  constraint horizontal L6
  constraint vertical L7
  constraint horizontal L8
  constraint vertical L9
  constraint coincident L2.start L5.end
  measures "d259" distance of L2.start L6.end
extrude "Extrude53" add sketch "Sketch49" along normal blind 3 contours L2 L4 L5 L6 L7 L8 L9 bodies 1
sketch "Sketch50" plane through (0, -12.5, 0) normal (0, -1, 0) x (1, 0, 0)
  line L0 (50, 0) -> (50, 90)
  arc A0 (50, 90) -> (20, 120) centre (20, 90) ccw
  line L1 (20, 120) -> (-20, 120)
  arc A1 (-20, 120) -> (-50, 90) centre (-20, 90) ccw
  line L2 (-50, 90) -> (-53, 90)
  line L3 (-53, 90) -> (-53, 0)
  line L4 (-53, 0) -> (50, 0)
  circle A2 centre (-0.0025, 70) radius 47.5
  circle A3 centre (-40, 6) radius 2.5
  circle A4 centre (-37.5, 32.5005) radius 3.5
  circle A5 centre (37.5, 32.5005) radius 3.5
  circle A6 centre (-37.5, 107.5005) radius 3.5
  circle A7 centre (37.5, 107.5005) radius 3.5
  line L5 (-50, 90) -> (-58, 90)
  line L6 (-58, 90) -> (-58, 0)
  line L7 (-58, 0) -> (-50, 0)
  line L8 (-50, 0) -> (-50, 90)
  constraint horizontal L5
  constraint vertical L6
  constraint horizontal L7
  constraint vertical L8
  constraint coincident A1.end L2.start
extrude "Extrude54" add sketch "Sketch50" along normal blind 3 contours L2 L3 L4 L5 L7 L8 | L3 L5 L6 L7 bodies 1
sketch "Sketch51" plane through (0, -12.5, 0) normal (0, 1, 0) x (-1, 0, 0)
  line L0 (53, 90) -> (53, 0)
  line L1 (53, 0) -> (58, 0)
  line L2 (58, 0) -> (58, 90)
  line L3 (58, 90) -> (53, 90)
  line L4 (57.5, 90) -> (55.5, 90)
  line L5 (55.5, 90) -> (55.5, 0)
  line L6 (55.5, 0) -> (57.5, 0)
  line L7 (57.5, 0) -> (57.5, 90)
  dimension "d264" = 0.5
  constraint horizontal L4
  constraint vertical L5
  constraint horizontal L6
  constraint vertical L7
  constraint coincident L1 L5.end
  constraint coincident L3 L4.start
  measures "d264" distance of L2 L7
extrude "Extrude55" add sketch "Sketch51" along normal blind 2 contours L1 L3 L4 L5 L6 L7 bodies 1
sketch "Sketch52" plane through (-50, 0, 0) normal (-1, 0, 0) x (0, -1, 0)
  line L0 (10.5, 0) -> (10.5, 90)
  line L1 (10.5, 90) -> (-12.5, 90)
  line L2 (-12.5, 90) -> (-12.5, 0)
  line L3 (-12.5, 0) -> (10.5, 0)
  line L4 (7.5, 30) -> (-7.5, 30)
  arc A0 (-7.5, 35) -> (-7.5, 30) centre (-7.5, 32.5) ccw
  line L5 (-7.5, 35) -> (7.5, 35)
  arc A1 (7.5, 30) -> (7.5, 35) centre (7.5, 32.5) ccw
  line L6 (-12.5, 90) -> (-10.5, 90)
  line L7 (-10.5, 90) -> (-10.5, 0)
  line L8 (-10.5, 0) -> (-12.5, 0)
  line L9 (-12.5, 0) -> (-12.5, 90)
  dimension "d267" = 2
  constraint perpendicular L6 L7
  constraint parallel L6 L8
  constraint parallel L7 L9
  constraint perpendicular L2 L6
  constraint coincident L1.end L2.start
  measures "d267" distance of L1.end L6.end
extrude "Extrude56" add sketch "Sketch52" along normal blind 3 contours L1 L2 L3 L6 L7 L8 L9 bodies 1